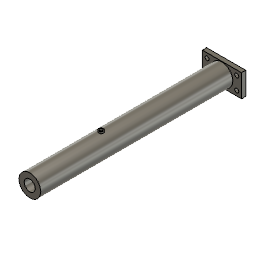
Measurement+Tube (Autodesk Fusion 360 design; units mm, degrees)
Autodesk Fusion 360 part; units mm, degrees
sketch "Sketch1" plane through (0, 0, 0) normal (0, 0, 1) x (1, 0, 0)
  circle A0 centre (0, 0) radius 6.375
  circle A1 centre (0, 0) radius 12.5
  dimension "d1" = 25
  dimension "d2" = 12.75
  constraint coincident A0.centre A1.centre
  measures "d1" diameter of A1
  measures "d2" diameter of A0
extrude "Extrude1" add sketch "Sketch1" along normal blind 225 contours A0 | A1
extrude "Extrude19" cut sketch "Sketch1" along normal up to surface (225 mm away) contours A0
sketch "Sketch22" plane through (0, 0, 0) normal (0, 0, 1) x (1, 0, 0)
  line L0 (22.5, 13) -> (-22.5, 13)
  line L1 (-22.5, 13) -> (-22.5, -13)
  line L2 (-22.5, -13) -> (22.5, -13)
  line L3 (22.5, -13) -> (22.5, 13)
  circle A0 centre (0, 0) radius 6.375 construction
  circle A1 centre (0, 0) radius 12.5 construction
  line L4 (0, 0) -> (22.5, 0) construction
  line L5 (0, 0) -> (-22.5, 0) construction
  circle A2 centre (0, 0) radius 12.5
  circle A3 centre (17, 7.5) radius 2.25
  circle A4 centre (-17, 7.5) radius 2.25
  circle A5 centre (-17, -7.5) radius 2.25
  circle A6 centre (17, -7.5) radius 2.25
  point P0 (12.5, 0)
  point P1 (-12.5, 0)
  dimension "d150" = 10
  dimension "d151" = 10
  dimension "d152" = 13
  dimension "d155" = 4.5
  dimension "d156" = 17
  dimension "d157" = 17
  dimension "d158" = 17
  dimension "d159" = 17
  dimension "d160" = 4.5
  dimension "d161" = 4.5
  dimension "d162" = 4.5
  dimension "d163" = 7.5
  dimension "d164" = 7.5
  dimension "d165" = 7.5
  dimension "d166" = 7.5
  constraint horizontal L0
  constraint vertical L1
  constraint horizontal L2
  constraint vertical L3
  constraint coincident A0.centre A1.centre
  constraint midpoint L3 L4.end
  constraint horizontal L4
  constraint coincident A1 P0
  constraint coincident L4 P0
  constraint midpoint L1 L5.end
  constraint coincident A1 P1
  constraint coincident L5 P1
  constraint coincident P0 A2
  measures "d150" distance of L4.end P0
  measures "d151" distance of L5.end P1
  measures "d152" distance of L0 A0.centre
  measures "d155" diameter of A3
  measures "d156" horizontal distance of A0.centre A3.centre
  measures "d157" horizontal distance of A0.centre A4.centre
  measures "d158" horizontal distance of A0.centre A6.centre
  measures "d159" horizontal distance of A0.centre A5.centre
  measures "d160" diameter of A4
  measures "d161" diameter of A6
  measures "d162" diameter of A5
  measures "d163" distance of L4 A3.centre
  measures "d164" distance of L5 A4.centre
  measures "d165" distance of L4 A6.centre
  measures "d166" distance of L5 A5.centre
extrude "Mount Holes" add sketch "Sketch22" along normal blind 5
ref_plane "WorkPlane4" through (0, 6.4, 0) normal (0, 1, 0) x (0, 0, 1)
sketch "Sketch21" plane through (0, 6.4, 0) normal (0, 1, 0) x (1, 0, 0)
  circle A0 centre (0, -143.363) radius 1.7
  circle A1 centre (0, -143.363) radius 2.7
  line L0 (-12.5, -225) -> (12.5, -225)
  line L1 (22.5, 0) -> (-22.5, 0) construction
  line L2 (-22.5, 0) -> (-22.5, -5) construction
  line L3 (-22.5, -5) -> (22.5, -5) construction
  line L4 (22.5, -5) -> (22.5, 0) construction
  line L5 (0, -5) -> (0, -225) construction
  dimension "d137" = 3.4
  dimension "d138" = 5.4
  dimension "d167" = 81.637
  constraint concentric A0 A1
  constraint midpoint L3 L5.start
  constraint midpoint L0 L5.end
  constraint coincident A0.centre L5
  measures "d137" diameter of A0
  measures "d138" diameter of A1
  measures "d167" distance of A0.centre L0
extrude "Extrude17" add sketch "Sketch21" along normal blind 8
extrude "Extrude18" cut sketch "Sketch21" along normal blind 8 and the other way blind 2 contours A0
equation "d5 = 12.8 mm"
equation "d20 = 0.105 in"
equation "d22 = d20"
equation "d29 = 2.5 in"
equation "d129 = 7.5 mm"
equation "d136 = d5 / 2"
equation "d138 = d137 + 2 mm"
equation "d151 = d150"
equation "d157 = d156"
equation "d158 = d156"
equation "d159 = d156"
equation "d160 = d155"
equation "d161 = d155"
equation "d162 = d155"
equation "d164 = d163"
equation "d165 = d163"
equation "d166 = d163"
equation "d50 = d48 / 2"
equation "d51 = d50"
equation "d52 = d53"
equation "d53 = d46 / 2"
equation "d54 = 4.25 mm"
equation "d55 = d54"
equation "d56 = -d45"
equation "d58 = 4.5 mm"
equation "d59 = d58"
equation "d64 = d67"
equation "d67 = 154.736 mm"
equation "d70 = d67"
equation "d110 = d26 / 2"
equation "d111 = d16 / 2"
equation "d115 = -d29"
equation "d119 = -d29"
equation "d127 = 17 mm"
equation "d128 = d127"
equation "d130 = d129"
equation "d131 = 4.25 mm"
equation "d132 = d131"
